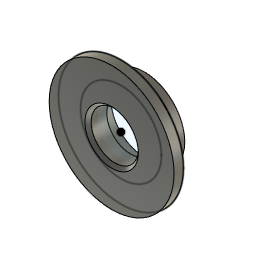
BASF Spool v1 (Autodesk Fusion 360 design; units mm, degrees)
Autodesk Fusion 360 part; units mm, degrees
sketch "Sketch1" plane through (0, 0, 0) normal (0, 1, 0) x (1, 0, 0)
  circle A0 centre (0, 0) radius 25.875
  circle A1 centre (0, 0) radius 40
  dimension "d1" = 51.75
  dimension "d2" = 80
  constraint coincident A0.centre A1.centre
  measures "d1" diameter of A0
  measures "d2" diameter of A1
extrude "Extrude1" add sketch "Sketch1" along normal blind 15 contours A0
extrude "Extrude2" add sketch "Sketch1" against normal blind 6 contours A0 | A1
sketch "Sketch2" plane through (0, 15, 0) normal (0, 1, 0) x (-1, 0, 0)
  circle A0 centre (0, 0) radius 25.875
  circle A1 centre (0, 0) radius 15.125
  dimension "d7" = 30.25
  constraint coincident A0.centre A1.centre
  measures "d7" diameter of A1
extrude "Extrude3" cut sketch "Sketch2" against normal blind 77.834 contours A1
sketch "Sketch3" plane through (0, 15, 0) normal (0, 1, 0) x (-1, 0, 0)
  circle A0 centre (0, 0) radius 15.125
  circle A1 centre (0, 0) radius 25.875
  circle A2 centre (0, 0) radius 21.5
  dimension "d10" = 43
  constraint concentric A0 A2
  measures "d10" diameter of A2
extrude "Extrude4" cut sketch "Sketch3" against normal blind 9 contours A2
chamfer "Chamfer1" distance 2 angle 45 1 edges at (14.1015, -6, -5.4694)
